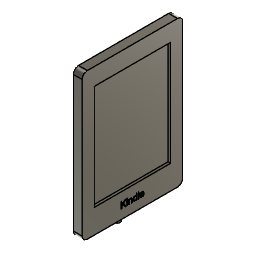
KindleHolder v4 (Autodesk Fusion 360 archive; units mm, degrees)
design "Kindle"
Autodesk Fusion 360 part; units mm, degrees
sketch "KindleSketch1" plane through (0, 0, 0) normal (1, 0, 0) x (0, 1, 0)
  line L0 (0, 35) -> (117, 35)
  line L1 (117, 35) -> (117, -135)
  line L2 (117, -135) -> (0, -135)
  line L3 (0, -135) -> (0, 35)
  dimension "d1" = 117
  dimension "d2" = 170
  constraint horizontal L0
  constraint vertical L1
  constraint horizontal L2
  constraint vertical L3
  measures "d1" distance of L0.start L0.end
  measures "d2" distance of L0.start L2.end
extrude "Extrude1" add sketch "KindleSketch1" along normal blind 10.3
sketch "KindleSketch2" plane through (0, 0, -135) normal (0, 0, -1) x (1, 0, 0)
  line L0 (0, 0) -> (0, -117)
  line L1 (0, -117) -> (10.3, -117)
  line L2 (10.3, -117) -> (10.3, 0)
  line L3 (10.3, 0) -> (0, 0)
  line L4 (5.15, 0) -> (5.15, -41.5)
  circle A0 centre (5.15, -45.5) radius 4
  line L5 (5.15, -117) -> (5.15, -75)
  line L6 (5.15, -75) -> (3.65, -75)
  line L7 (3.65, -75) -> (3.65, -67.5)
  line L8 (3.65, -67.5) -> (5.15, -67.5)
  line L9 (5.15, -67.5) -> (5.15, -75)
  line L10 (5.15, -75) -> (6.65, -75)
  line L11 (6.65, -75) -> (6.65, -67.5)
  line L12 (6.65, -67.5) -> (5.15, -67.5)
  line L13 (5.15, -67.5) -> (5.15, -75)
  dimension "d5" = 41.5
  dimension "d6" = 8
  dimension "d9" = 42
  dimension "d10" = 7.5
  dimension "d11" = 1.5
  dimension "d12" = 7.5
  constraint vertical L4
  constraint midpoint L3 L4.start
  constraint coincident L4.end A0
  constraint vertical L5
  constraint midpoint L1 L5.start
  constraint horizontal L6
  constraint vertical L7
  constraint horizontal L8
  constraint vertical L9
  constraint horizontal L10
  constraint vertical L11
  constraint horizontal L12
  constraint vertical L13
  measures "d5" distance of L4.start L4.end
  measures "d6" diameter of A0
  measures "d9" distance of L5.start L5.end
  measures "d10" distance of L5.end L8.end
  measures "d11" distance of L5.end L6.end
  measures "d12" distance of L5.end L8.end
extrude "Extrude3" add sketch "KindleSketch2" along normal blind 0.5 contours L6 L7 L8 L9 L13 | L9 L10 L11 L12 L13
extrude "Extrude2" add sketch "KindleSketch2" along normal blind 3.5 contours A0
sketch "KindleSketch3" plane through (10.3, 0, 0) normal (1, 0, 0) x (0, 1, 0)
  line L0 (0, -135) -> (117, -135)
  line L1 (117, -135) -> (117, 35)
  line L2 (117, 35) -> (0, 35)
  line L3 (0, 35) -> (0, -135)
  line L4 (45.3067, -124.4813) -> (71.9571, -124.4813) construction
  line L5 (71.9571, -124.4813) -> (71.9571, -114.4813) construction
  line L6 (71.9571, -114.4813) -> (45.3067, -114.4813) construction
  line L7 (45.3067, -114.4813) -> (45.3067, -124.4813) construction
  line L8 (0, 35) -> (117, 35)
  line L9 (117, 35) -> (117, 15)
  line L10 (117, 15) -> (0, 15)
  line L11 (0, 15) -> (0, 35)
  line L12 (0, 35) -> (14, 35)
  line L13 (14, 35) -> (14, -135)
  line L14 (14, -135) -> (0, -135)
  line L15 (0, -135) -> (0, 35)
  line L16 (117, 35) -> (103, 35)
  line L17 (103, 35) -> (103, -135)
  line L18 (103, -135) -> (117, -135)
  line L19 (117, -135) -> (117, 35)
  line L20 (0, -135) -> (117, -135)
  line L21 (117, -135) -> (117, -107)
  line L22 (117, -107) -> (0, -107)
  line L23 (0, -107) -> (0, -135)
  dimension "d17" = 117
  dimension "d18" = 20
  dimension "d19" = 14
  dimension "d20" = 170
  dimension "d21" = 170
  dimension "d22" = 14
  dimension "d23" = 117
  dimension "d24" = 28
  text T0 "Kindle" font "Arial" height 10 align ink ink in box 0 x 0 at (45.3067, -124.4813) x (1, 0) y (0, 1) spacing 1 height is em
  constraint perpendicular L4 L5
  constraint parallel L4 L6
  constraint parallel L5 L7
  constraint horizontal L8
  constraint vertical L9
  constraint horizontal L10
  constraint vertical L11
  constraint coincident L2.end L3.start
  constraint horizontal L12
  constraint vertical L13
  constraint horizontal L14
  constraint vertical L15
  constraint horizontal L16
  constraint vertical L17
  constraint horizontal L18
  constraint vertical L19
  constraint horizontal L20
  constraint vertical L21
  constraint horizontal L22
  constraint vertical L23
  constraint coincident L0.start L3.end
  measures "d17" distance of L2.end L1.end
  measures "d18" distance of L2.end L10.end
  measures "d19" distance of L2.end L12.end
  measures "d20" distance of L2.end L0.start
  measures "d21" distance of L1.end L0.end
  measures "d22" distance of L1.end L16.end
  measures "d23" distance of L0.start L0.end
  measures "d24" distance of L0.start L22.end
extrude "Extrude5" cut sketch "KindleSketch3" against normal blind 3 contours L10 L13 L17 L22
extrude "Extrude4" cut sketch "KindleSketch3" against normal blind 1 text T0
fillet "Fillet1" radius 6 4 edges at (5.15, 0, -135) (5.15, 117, -135) (5.15, 0, 35) (5.15, 117, 35)
named bodies: "Kindle"
